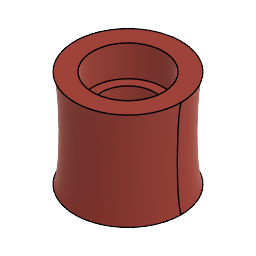
BearingSleeve_v8 (Autodesk Fusion 360 design; units mm, degrees)
Autodesk Fusion 360 part; units mm, degrees
sketch "Sketch1" plane through (0, 0, 0) normal (0, 0, 1) x (1, 0, 0)
  circle A0 centre (0, 0) radius 4
  circle A1 centre (0, 0) radius 6
  circle A2 centre (0, 0) radius 3
  dimension "d1" = 8
  dimension "d2" = 12
  dimension "d3" = 6
  constraint coincident A0.centre A1.centre
  constraint concentric A0 A2
  measures "d1" diameter of A0
  measures "d2" diameter of A1
  measures "d3" diameter of A2
extrude "Extrude1" add sketch "Sketch1" along normal blind 4 contours A1
extrude "Extrude2" add sketch "Sketch1" along normal blind 7.5 from surface at 4 contours A0 | A1
extrude "Extrude3" cut sketch "Sketch1" along normal blind 4 from surface at 8 contours A0
move_face "OffsetFaces1" offset -0.5 1 faces at (5.2961, -0.4968, 0)
sketch "Sketch2" plane through (0, 0, 0) normal (0, 1, 0) x (1, 0, 0)
  line L0 (6, -0.5) -> (6, -11.5)
  spline S0 degree 5 poles (6, -11.5) (5.9399, -11.2998) (5.8306, -10.7774) (5.6989, -9.6281) (5.5847, -7.5081) (5.5492, -4.5095) (5.6313, -2.3856) (5.7779, -1.2306) (5.9188, -0.7031) (6, -0.5) knots 0 0 0 0 0 0 0.2 0.4 0.6 0.8 1 1 1 1 1 1
  line L1 (5.8, -1) -> (6.2, 0)
  line L2 (6.15, -12) -> (5.85, -11)
  line L3 (6, -11.5) -> (6, -0.5)
  constraint vertical L0
  constraint midpoint L0.start L1
  constraint midpoint L0.end L2
revolve "Revolve1" cut sketch "Sketch2" angle 360 about axis through (0, 0, 1.75) along (0, 0, 1)
equation "d7 = 8 mm - 0.5 mm"
